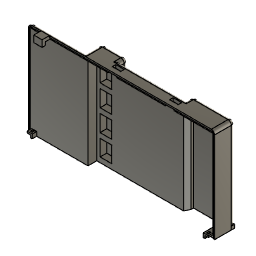
lcd_back (Autodesk Fusion 360 design; units mm, degrees)
Autodesk Fusion 360 part; units mm, degrees
note: some values were not read from the file. Set by a fixed rule: which sketch regions a step uses.
sketch "Szkic1" plane through (0, 0, 0) normal (0, 0, 1) x (1, 0, 0)
  line L0 (0, 0) -> (68.2, 0)
  line L1 (68.2, 0) -> (68.2, 10.6)
  line L2 (68.2, 10.6) -> (176, 10.6)
  line L3 (219, 19.6) -> (219, 23.4)
  line L4 (219, 23.4) -> (62.2, 23.4)
  line L5 (62.2, 23.4) -> (62.2, 3.4)
  line L6 (62.2, 3.4) -> (0, 3.4)
  line L7 (0, 3.4) -> (0, 0)
  circle A0 centre (168, 18.6) radius 1.6
  circle A1 centre (96.5, 18.6) radius 1.6
  line L8 (176, 10.6) -> (176, 19.6)
  line L9 (176, 19.6) -> (219, 19.6)
  dimension "d1" = 62.2
  dimension "d2" = 3.4
  dimension "d3" = 219
  dimension "d4" = 6
  dimension "d5" = 20
  dimension "d6" = 3.2
  dimension "d7" = 3.2
  dimension "d8" = 4.8
  dimension "d9" = 51
  dimension "d10" = 122.5
  dimension "d12" = 12.8
  dimension "d13" = 8
  dimension "d14" = 3.8
  constraint coincident L0.start L7.end
  constraint horizontal L0
  constraint perpendicular L0 L1
  constraint perpendicular L1 L2
  constraint perpendicular L2 L3
  constraint perpendicular L1 L4
  constraint perpendicular L4 L5
  constraint perpendicular L1 L6
  constraint perpendicular L0 L7
  constraint horizontal A0.centre A1.centre
  constraint perpendicular L2 L8
  constraint perpendicular L8 L9
  measures "d1" distance of L5.end L6.end
  measures "d2" distance of L0 L6
  measures "d3" distance of L0.start L3
  measures "d4" distance of L1 L5
  measures "d5" distance of L4 L6
  measures "d6" diameter of A0
  measures "d7" diameter of A1
  measures "d8" distance of L4 A0.centre
  measures "d9" distance of L3 A0.centre
  measures "d10" distance of L3 A1.centre
  measures "d12" distance of L2 L4
  measures "d13" distance of A0.centre L8
  measures "d14" distance of L4 L9
extrude "Wyciągnięcie proste1" add sketch "Szkic1" along normal blind 4
sketch "Szkic2" plane through (0, 0, 4) normal (0, 0, 1) x (-1, 0, 0)
  circle A0 centre (-168, -18.6) radius 1.6
  circle A1 centre (-96.5, -18.6) radius 1.6
  line L0 (-176, -19.6) -> (-219, -19.6)
  line L1 (-219, -19.6) -> (-219, -23.4)
  line L2 (-219, -23.4) -> (-62.2, -23.4)
  line L3 (-62.2, -23.4) -> (-62.2, -3.4)
  line L4 (-62.2, -3.4) -> (0, -3.4)
  line L5 (0, -3.4) -> (0, 0)
  line L6 (0, 0) -> (-68.2, 0)
  line L7 (-68.2, 0) -> (-68.2, -10.6)
  line L8 (-68.2, -10.6) -> (-176, -10.6)
  line L9 (-176, -10.6) -> (-176, -19.6)
  circle A2 centre (-96.5, -18.6) radius 3
  circle A3 centre (-168, -18.6) radius 3
  dimension "d17" = 6
  dimension "d18" = 6
  constraint concentric A1 A2
  constraint concentric A0 A3
  measures "d17" diameter of A2
  measures "d18" diameter of A3
extrude "Wyciągnięcie proste2" cut sketch "Szkic2" against normal blind 2 contours A2 | A3
sketch "Szkic3" plane through (0, 0, 4) normal (0, 0, 1) x (-1, 0, 0)
  circle A0 centre (-96.5, -18.6) radius 3
  circle A1 centre (-168, -18.6) radius 3
  line L0 (-176, -19.6) -> (-219, -19.6)
  line L1 (-219, -19.6) -> (-219, -23.4)
  line L2 (-219, -23.4) -> (-62.2, -23.4)
  line L3 (-62.2, -23.4) -> (-62.2, -3.4)
  line L4 (-62.2, -3.4) -> (0, -3.4)
  line L5 (0, -3.4) -> (0, 0)
  line L6 (0, 0) -> (-68.2, 0)
  line L7 (-68.2, 0) -> (-68.2, -10.6)
  line L8 (-68.2, -10.6) -> (-176, -10.6)
  line L9 (-176, -10.6) -> (-176, -19.6)
  line L10 (0, -3.4) -> (-62.2, -3.4)
  line L11 (-62.2, -23.4) -> (-62.2, -3.4)
  line L12 (-62.2, -23.4) -> (-92.5, -23.4)
  line L13 (-92.5, -14.6) -> (-172, -14.6)
  line L14 (-172, -14.6) -> (-172, -23.4)
  line L15 (-172, -23.4) -> (-219, -23.4)
  line L16 (-219, -23.4) -> (-219, -19.6)
  line L17 (-219, -19.6) -> (-176, -19.6)
  line L18 (-176, -19.6) -> (-176, -10.6)
  line L19 (-176, -10.6) -> (-68.2, -10.6)
  line L20 (-68.2, -10.6) -> (-68.2, 0)
  line L21 (-68.2, 0) -> (0, 0)
  line L22 (0, -3.4) -> (0, 0)
  line L23 (-92.5, -14.6) -> (-92.5, -23.4)
  dimension "d21" = 4
  dimension "d22" = 4
  dimension "d24" = 4
  constraint coincident L4.end L5.start
  constraint coincident L3.end L4.start
  constraint coincident L2.end L3.start
  constraint coincident L2 L12.end
  constraint perpendicular L3 L12
  constraint parallel L8 L13
  constraint coincident L2 L14.end
  constraint perpendicular L2 L14
  constraint coincident L1.end L2.start
  constraint coincident L0.end L1.start
  constraint coincident L0.start L9.end
  constraint coincident L8.end L9.start
  constraint coincident L7.end L8.start
  constraint coincident L6.end L7.start
  constraint coincident L5.end L6.start
  constraint perpendicular L12 L23
  constraint coincident L13.end L14.start
  measures "d21" distance of A0.centre L23
  measures "d22" distance of A1.centre L14
  measures "d24" distance of A0.centre L13
extrude "Wyciągnięcie proste3" add sketch "Szkic3" along normal blind 105.486 contours L0 L1 L2 L3 L4 L5 L6 L7 L8 L9 L10 L11 L12 L13 L14 L15 L16 L17 L18 L19 L20 L21 L22 L23
sketch "Szkic4" plane through (0, 0, 109.486) normal (0, 0, 1) x (-1, 0, 0)
  line L0 (-172, -14.6) -> (-92.5, -14.6)
  line L1 (-92.5, -14.6) -> (-92.5, -23.4)
  line L2 (-92.5, -23.4) -> (-62.2, -23.4)
  line L3 (-62.2, -23.4) -> (-62.2, -3.4)
  line L4 (-62.2, -3.4) -> (0, -3.4)
  line L5 (0, -3.4) -> (0, 0)
  line L6 (0, 0) -> (-68.2, 0)
  line L7 (-68.2, 0) -> (-68.2, -10.6)
  line L8 (-68.2, -10.6) -> (-176, -10.6)
  line L9 (-176, -10.6) -> (-176, -19.6)
  line L10 (-176, -19.6) -> (-219, -19.6)
  line L11 (-219, -19.6) -> (-219, -23.4)
  line L12 (-219, -23.4) -> (-172, -23.4)
  line L13 (-172, -23.4) -> (-172, -14.6)
  line L14 (0, -3.4) -> (-62.2, -3.4)
  line L15 (-62.2, -3.4) -> (-62.2, -23.4)
  line L16 (-62.2, -23.4) -> (-92.5, -23.4)
  line L17 (-92.5, -23.4) -> (-92.5, -14.6)
  line L18 (-92.5, -14.6) -> (-172, -14.6)
  line L19 (-172, -14.6) -> (-172, -23.4)
  line L20 (-172, -23.4) -> (-219, -23.4)
  line L21 (-219, -23.4) -> (-219, -0.0002)
  line L22 (-219, -0.0002) -> (0, 0)
  line L23 (0, 0) -> (0, -3.4)
  constraint coincident L4.end L5.start
  constraint coincident L3.end L4.start
  constraint coincident L2.end L3.start
  constraint coincident L1.end L2.start
  constraint coincident L0.end L1.start
  constraint coincident L0.start L13.end
  constraint coincident L12.end L13.start
  constraint coincident L11.end L12.start
  constraint coincident L5.end L6.start
  constraint perpendicular L21 L22
  constraint perpendicular L22 L23
extrude "Wyciągnięcie proste4" add sketch "Szkic4" along normal blind 4
sketch "Szkic5" plane through (0, 0, 113.486) normal (0, 0, 1) x (-1, 0, 0)
  line L0 (0, 0) -> (-219, -0.0002)
  line L1 (-219, -0.0002) -> (-219, -23.4)
  line L2 (-219, -23.4) -> (-172, -23.4)
  line L3 (-172, -23.4) -> (-172, -14.6)
  line L4 (-172, -14.6) -> (-92.5, -14.6)
  line L5 (-92.5, -14.6) -> (-92.5, -23.4)
  line L6 (-92.5, -23.4) -> (-62.2, -23.4)
  line L7 (-62.2, -23.4) -> (-62.2, -3.4)
  line L8 (-62.2, -3.4) -> (0, -3.4)
  line L9 (0, -3.4) -> (0, 0)
  line L10 (-92.5, -9.2001) -> (-102.7, -9.2001)
  line L11 (-102.7, -9.2001) -> (-102.7, -5.0001)
  line L12 (-102.7, -5.0001) -> (-92.5, -5.0001)
  line L13 (-92.5, -5.0001) -> (-92.5, -9.2001)
  line L14 (-161.8, -9.2001) -> (-172, -9.2001)
  line L15 (-172, -9.2001) -> (-172, -5.0001)
  line L16 (-172, -5.0001) -> (-161.8, -5.0001)
  line L17 (-161.8, -5.0001) -> (-161.8, -9.2001)
  dimension "d29" = 4.2
  dimension "d30" = 10.2
  dimension "d31" = 4.2
  dimension "d32" = 10.2
  dimension "d33" = 5
  dimension "d34" = 5
  constraint horizontal L10
  constraint vertical L11
  constraint horizontal L12
  constraint vertical L13
  constraint horizontal L14
  constraint vertical L15
  constraint horizontal L16
  constraint vertical L17
  constraint vertical L3.end L14.end
  constraint vertical L4.end L10.start
  measures "d29" distance of L10.start L12.end
  measures "d30" distance of L10.start L10.end
  measures "d31" distance of L14.end L15.end
  measures "d32" distance of L14.start L14.end
  measures "d33" distance of L0 L12
  measures "d34" distance of L0 L16
extrude "Wyciągnięcie proste5" cut sketch "Szkic5" against normal blind 5 contours L10 L11 L12 L13 | L14 L15 L16 L17
sketch "Szkic6" plane through (0, 0, 109.486) normal (0, 0, -1) x (1, 0, 0)
  line L0 (102.7, -5.0001) -> (102.7, -9.2001)
  line L1 (102.7, -9.2001) -> (92.5, -9.2001)
  line L2 (92.5, -9.2001) -> (92.5, -5.0001)
  line L3 (92.5, -5.0001) -> (102.7, -5.0001)
  line L4 (172, -5.0001) -> (172, -9.2001)
  line L5 (172, -9.2001) -> (161.8, -9.2001)
  line L6 (161.8, -9.2001) -> (161.8, -5.0001)
  line L7 (161.8, -5.0001) -> (172, -5.0001)
  line L8 (68.2, -0.0001) -> (68.2, -10.6)
  line L9 (68.2, -10.6) -> (176, -10.6)
  line L10 (176, -10.6) -> (176, -19.6)
  line L11 (176, -19.6) -> (219, -19.6)
  line L12 (219, -19.6) -> (219, -0.0002)
  line L13 (219, -0.0002) -> (68.2, -0.0001)
  line L14 (92.5, -5.0001) -> (102.7, -5.0001)
  line L15 (102.7, -5.0001) -> (102.7, -0.0001)
  line L16 (102.7, -0.0001) -> (92.5, -0.0001)
  line L17 (92.5, -0.0001) -> (92.5, -5.0001)
  line L18 (161.8, -5.0001) -> (172, -5.0001)
  line L19 (172, -5.0001) -> (172, -0.0001)
  line L20 (172, -0.0001) -> (161.8, -0.0001)
  line L21 (161.8, -0.0001) -> (161.8, -5.0001)
  constraint horizontal L14
  constraint vertical L15
  constraint horizontal L16
  constraint vertical L17
  constraint coincident L2.end L3.start
  constraint horizontal L18
  constraint vertical L19
  constraint horizontal L20
  constraint vertical L21
  constraint coincident L6.end L7.start
  constraint coincident L0.start L3.end
  constraint coincident L13 L15.end
  constraint coincident L13 L19.end
  constraint coincident L4.start L19
extrude "Wyciągnięcie proste6" cut sketch "Szkic6" against normal blind 2 contours L3 L13 L14 L15 L16 L17 | L7 L13 L18 L19 L20 L21
sketch "Szkic7" plane through (0, 0, 0) normal (-1, 0, 0) x (0, -1, 0)
  line L0 (-3.4, 0) -> (0, 0)
  line L1 (0, 0) -> (0, 109.486)
  line L2 (0, 109.486) -> (0, 113.486)
  line L3 (0, 113.486) -> (-3.4, 113.486)
  line L4 (-3.4, 113.486) -> (-3.4, 0)
  line L5 (-3.4, 113.486) -> (0, 113.486)
  line L6 (0, 113.486) -> (0, 0)
  line L7 (0, 0) -> (-3.4, 0)
  line L8 (-3.4, 0) -> (-3.4, 113.486)
  constraint horizontal L5
  constraint vertical L6
  constraint horizontal L7
  constraint vertical L8
  constraint coincident L0.end L1.start
  constraint coincident L3.end L4.start
extrude "Wyciągnięcie proste7" add sketch "Szkic7" along normal blind 2.8
sketch "Szkic8" plane through (219, 0.0002, 0) normal (1, 0.000001, 0) x (-0.000001, 1, 0)
  line L0 (19.5998, 0) -> (23.3998, 0)
  line L1 (23.3998, 0) -> (23.3998, 113.486)
  line L2 (23.3998, 113.486) -> (0, 113.486)
  line L3 (0, 113.486) -> (0, 109.486)
  line L4 (0, 109.486) -> (19.5998, 109.486)
  line L5 (19.5998, 109.486) -> (19.5998, 0)
  line L6 (23.3998, 113.486) -> (0, 113.486)
  line L7 (0, 113.486) -> (0, 0)
  line L8 (0, 0) -> (23.3998, 0)
  line L9 (23.3998, 0) -> (23.3998, 113.486)
  constraint horizontal L6
  constraint vertical L7
  constraint horizontal L8
  constraint vertical L9
  constraint coincident L7.end L8.start
  constraint coincident L1.end L2.start
extrude "Wyciągnięcie proste8" add sketch "Szkic8" along normal blind 2.8
sketch "Szkic9" plane through (0, 0, 113.486) normal (0, 0, 1) x (-1, 0, 0)
  line L0 (-102.7, -9.2001) -> (-102.7, -5.0001)
  line L1 (-102.7, -5.0001) -> (-92.5, -5.0001)
  line L2 (-92.5, -5.0001) -> (-92.5, -9.2001)
  line L3 (-92.5, -9.2001) -> (-102.7, -9.2001)
  line L4 (-172, -9.2001) -> (-172, -5.0001)
  line L5 (-172, -5.0001) -> (-161.8, -5.0001)
  line L6 (-161.8, -5.0001) -> (-161.8, -9.2001)
  line L7 (-161.8, -9.2001) -> (-172, -9.2001)
  line L8 (0, 0) -> (-221.8, -0.0002)
  line L9 (-221.8, -0.0002) -> (-221.8, -23.4)
  line L10 (-221.8, -23.4) -> (-219, -23.4)
  line L11 (-219, -23.4) -> (-172, -23.4)
  line L12 (-172, -23.4) -> (-172, -14.6)
  line L13 (-172, -14.6) -> (-92.5, -14.6)
  line L14 (-92.5, -14.6) -> (-92.5, -23.4)
  line L15 (-92.5, -23.4) -> (-62.2, -23.4)
  line L16 (-62.2, -23.4) -> (-62.2, -3.4)
  line L17 (-62.2, -3.4) -> (2.8, -3.4)
  line L18 (2.8, -3.4) -> (2.8, 0)
  line L19 (2.8, 0) -> (0, 0)
  line L20 (-12.2, 0) -> (-22.2, 0)
  line L21 (-22.2, 0) -> (-22.2, 9.4)
  line L22 (-22.2, 9.4) -> (-12.2, 9.4)
  line L23 (-12.2, 9.4) -> (-12.2, 0)
  dimension "d43" = 9.4
  dimension "d44" = 10
  dimension "d45" = 15
  constraint horizontal L20
  constraint vertical L21
  constraint horizontal L22
  constraint vertical L23
  constraint coincident L8 L20.end
  measures "d43" distance of L8 L22
  measures "d44" distance of L21 L23
  measures "d45" distance of L18 L23
extrude "Wyciągnięcie proste9" add sketch "Szkic9" against normal blind 4 contours L8 L20 L21 L22 L23
sketch "Szkic10" plane through (0, 0, 109.486) normal (0, 0, -1) x (1, 0, 0)
  line L0 (22.2, 9.4) -> (12.2, 9.4)
  line L1 (12.2, 9.4) -> (12.2, 0)
  line L2 (12.2, 0) -> (22.2, 0)
  line L3 (22.2, 0) -> (22.2, 9.4)
  line L4 (12.2, 9.4) -> (22.2, 9.4)
  line L5 (22.2, 9.4) -> (22.2, 5.4)
  line L6 (22.2, 5.4) -> (12.2, 5.4)
  line L7 (12.2, 5.4) -> (12.2, 9.4)
  dimension "d48" = 4
  constraint horizontal L4
  constraint vertical L5
  constraint horizontal L6
  constraint vertical L7
  constraint coincident L3 L5.end
  constraint coincident L0.end L1.start
  measures "d48" distance of L4 L6
extrude "Wyciągnięcie proste10" add sketch "Szkic10" along normal blind 4 contours L0 L1 L3 L4 L5 L6 L7
sketch "Szkic12" plane through (219, 0.0002, 0) normal (-1, -0.000001, 0) x (0.000001, -1, 0)
  line L0 (-19.5998, 109.486) -> (-19.5998, 0)
  line L1 (-19.5998, 0) -> (0, 0)
  line L2 (0, 0) -> (0, 109.486)
  line L3 (0, 109.486) -> (-19.5998, 109.486)
  line L4 (0, 0) -> (-19.5998, 0)
  line L5 (-19.5998, 0) -> (-19.5998, 5)
  line L6 (-19.5998, 5) -> (0, 5)
  line L7 (0, 5) -> (0, 0)
  dimension "d58" = 5
  constraint horizontal L4
  constraint vertical L5
  constraint horizontal L6
  constraint vertical L7
  constraint coincident L0 L5.end
  constraint coincident L1.end L2.start
  measures "d58" distance of L4 L6
extrude "Wyciągnięcie proste12" add sketch "Szkic12" along normal blind 6.3 contours L0 L1 L2 L4 L5 L6 L7
sketch "Szkic13" plane through (0, 0, 0) normal (0.000001, -1, 0) x (1, 0.000001, 0)
  line L0 (22.2, 113.486) -> (22.2, 109.486)
  line L1 (22.2, 109.486) -> (68.2, 109.486)
  line L2 (68.2, 109.486) -> (92.5, 109.486)
  line L3 (92.5, 109.486) -> (92.5, 111.486)
  line L4 (92.5, 111.486) -> (102.7, 111.486)
  line L5 (102.7, 111.486) -> (102.7, 109.486)
  line L6 (102.7, 109.486) -> (161.8, 109.486)
  line L7 (161.8, 109.486) -> (161.8, 111.486)
  line L8 (161.8, 111.486) -> (172, 111.486)
  line L9 (172, 111.486) -> (172, 109.486)
  line L10 (172, 109.486) -> (219, 109.486)
  line L11 (219, 109.486) -> (219, 5)
  line L12 (219, 5) -> (212.7, 5)
  line L13 (212.7, 5) -> (212.7, 0)
  line L14 (212.7, 0) -> (221.8, 0)
  line L15 (221.8, 0) -> (221.8, 113.486)
  line L16 (221.8, 113.486) -> (22.2, 113.486)
  line L17 (212.7, 0) -> (218.9, 0)
  line L18 (218.9, 0) -> (218.9, 5)
  line L19 (218.9, 5) -> (212.7, 5)
  line L20 (212.7, 5) -> (212.7, 0)
  dimension "d61" = 0.1
  constraint horizontal L17
  constraint vertical L18
  constraint horizontal L19
  constraint vertical L20
  constraint coincident L12 L18.end
  constraint coincident L13.end L14.start
  measures "d61" distance of L11 L18
extrude "Wyciągnięcie proste13" add sketch "Szkic13" along normal blind 5.4 contours L12 L13 L14 L17 L18 L19 L20
sketch "Szkic14" plane through (218.9, 0.0002, 0) normal (1, 0.000001, 0) x (-0.000001, 1, 0)
  line L0 (0, 0) -> (0, 5)
  line L1 (0, 5) -> (-5.4, 5)
  line L2 (-5.4, 5) -> (-5.4, 0)
  line L3 (-5.4, 0) -> (0, 0)
  line L4 (-5.4, 0) -> (0, 0)
  line L5 (0, 0) -> (0, 3.1)
  line L6 (0, 3.1) -> (-5.4, 3.1)
  line L7 (-5.4, 3.1) -> (-5.4, 0)
  dimension "d64" = 3.1
  constraint horizontal L4
  constraint vertical L5
  constraint horizontal L6
  constraint vertical L7
  constraint coincident L0 L5.end
  constraint coincident L2.end L3.start
  measures "d64" distance of L2.end L6.end
extrude "Wyciągnięcie proste14" cut sketch "Szkic14" against normal blind 4.2 contours L0 L2 L3 L4 L5 L6 L7
sketch "Szkic15" plane through (0, 0, 5) normal (0, 0, 1) x (-1, 0, 0)
  line L0 (-219, -0.0002) -> (-219, -19.6)
  line L1 (-219, -19.6) -> (-212.7, -19.6)
  line L2 (-212.7, -19.6) -> (-212.7, 5.3998)
  line L3 (-212.7, 5.3998) -> (-218.9, 5.3998)
  line L4 (-218.9, 5.3998) -> (-218.9, -0.0002)
  line L5 (-218.9, -0.0002) -> (-219, -0.0002)
  line L6 (-214.7, 0.1998) -> (-216.9, 0.1998)
  line L7 (-216.9, 0.1998) -> (-216.9, 3.3998)
  line L8 (-216.9, 3.3998) -> (-214.7, 3.3998)
  line L9 (-214.7, 3.3998) -> (-214.7, 0.1998)
  dimension "d67" = 2.2
  dimension "d68" = 3.2
  dimension "d69" = 2
  dimension "d70" = 2
  constraint horizontal L6
  constraint vertical L7
  constraint horizontal L8
  constraint vertical L9
  measures "d67" distance of L6.start L6.end
  measures "d68" distance of L6.end L7.end
  measures "d69" distance of L4 L7
  measures "d70" distance of L3 L8
extrude "Wyciągnięcie proste15" cut sketch "Szkic15" against normal blind 10 contours L6 L7 L8 L9
sketch "Szkic16" plane through (0, 0, 0) normal (0, -1, 0) x (1, 0, 0)
  line L0 (-2.8, 0) -> (68.2, 0)
  line L1 (68.2, 0) -> (68.2, 109.486)
  line L2 (68.2, 109.486) -> (22.2, 109.486)
  line L3 (22.2, 109.486) -> (12.2, 109.486)
  line L4 (12.2, 109.486) -> (0, 109.486)
  line L5 (0, 109.486) -> (0, 113.486)
  line L6 (0, 113.486) -> (-2.8, 113.486)
  line L7 (-2.8, 113.486) -> (-2.8, 0)
  line L8 (0.1, 0) -> (6.3, 0)
  line L9 (6.3, 0) -> (6.3, 5)
  line L10 (6.3, 5) -> (0.1, 5)
  line L11 (0.1, 5) -> (0.1, 0)
  dimension "d73" = 2.9
  dimension "d74" = 5
  dimension "d75" = 6.2
  constraint horizontal L8
  constraint vertical L9
  constraint horizontal L10
  constraint vertical L11
  constraint coincident L0 L8.start
  measures "d73" distance of L7 L11
  measures "d74" distance of L8.end L9.end
  measures "d75" distance of L9.end L10.end
extrude "Wyciągnięcie proste16" add sketch "Szkic16" along normal blind 5.4 contours L0 L8 L9 L10 L11
sketch "Szkic18" plane through (0.1, 0, 0) normal (-1, 0, 0) x (0, -1, 0)
  line L0 (0, 5) -> (0, 0)
  line L1 (0, 0) -> (5.4, 0)
  line L2 (5.4, 0) -> (5.4, 5)
  line L3 (5.4, 5) -> (0, 5)
  line L4 (5.4, 0) -> (-0.0002, 0)
  line L5 (-0.0002, 0) -> (-0.0002, 3.1)
  line L6 (-0.0002, 3.1) -> (5.4, 3.1)
  line L7 (5.4, 3.1) -> (5.4, 0)
  point P0 (-0.0002, 3.1)
  dimension "d80" = 3.1
  constraint horizontal L4
  constraint vertical L5
  constraint horizontal L6
  constraint vertical L7
  constraint coincident L1.end L2.start
  constraint coincident P0 L5.end
  measures "d80" distance of L1.end L6.end
extrude "Wyciągnięcie proste17" cut sketch "Szkic18" against normal blind 4.2 contours L0 L1 L2 L4 L5 L6 L7
sketch "Szkic19" plane through (0, 0, 5) normal (0, 0, 1) x (-1, 0, 0)
  line L0 (-6.3, 0) -> (-0.1, 0)
  line L1 (-0.1, 0) -> (-0.1, 5.4)
  line L2 (-0.1, 5.4) -> (-6.3, 5.4)
  line L3 (-6.3, 5.4) -> (-6.3, 0)
  line L4 (-2.1, 0.2) -> (-4.3, 0.2)
  line L5 (-4.3, 0.2) -> (-4.3, 3.4)
  line L6 (-4.3, 3.4) -> (-2.1, 3.4)
  line L7 (-2.1, 3.4) -> (-2.1, 0.2)
  dimension "d83" = 2.2
  dimension "d84" = 3.2
  dimension "d85" = 2
  dimension "d86" = 2
  constraint horizontal L4
  constraint vertical L5
  constraint horizontal L6
  constraint vertical L7
  measures "d83" distance of L4.start L4.end
  measures "d84" distance of L4.end L5.end
  measures "d85" distance of L2 L6
  measures "d86" distance of L1 L7
extrude "Wyciągnięcie proste18" cut sketch "Szkic19" against normal blind 10 contours L4 L5 L6 L7
sketch "Szkic20" plane through (0, 0, 0) normal (0.000001, -1, 0) x (1, 0.000001, 0)
  line L0 (218.9, 5) -> (218.9, 3.1)
  line L1 (218.9, 3.1) -> (214.7, 3.1)
  line L2 (214.7, 3.1) -> (214.7, 0)
  line L3 (214.7, 0) -> (221.8, 0)
  line L4 (221.8, 0) -> (221.8, 113.486)
  line L5 (221.8, 113.486) -> (22.2, 113.486)
  line L6 (22.2, 113.486) -> (22.2, 109.486)
  line L7 (22.2, 109.486) -> (68.2, 109.486)
  line L8 (68.2, 109.486) -> (92.5, 109.486)
  line L9 (92.5, 109.486) -> (92.5, 111.486)
  line L10 (92.5, 111.486) -> (102.7, 111.486)
  line L11 (102.7, 111.486) -> (102.7, 109.486)
  line L12 (102.7, 109.486) -> (161.8, 109.486)
  line L13 (161.8, 109.486) -> (161.8, 111.486)
  line L14 (161.8, 111.486) -> (172, 111.486)
  line L15 (172, 111.486) -> (172, 109.486)
  line L16 (172, 109.486) -> (219, 109.486)
  line L17 (219, 109.486) -> (219, 5)
  line L18 (219, 5) -> (218.9, 5)
  line L19 (22.2, 113.486) -> (221.8, 113.486)
  line L20 (221.8, 113.486) -> (221.8, 0)
  line L21 (221.8, 0) -> (220.55, 0)
  line L22 (220.55, 0) -> (220.55, 110.136)
  line L23 (219.05, 111.636) -> (22.2, 111.636)
  line L24 (22.2, 111.636) -> (22.2, 113.486)
  arc A0 (220.55, 110.136) -> (219.05, 111.636) centre (219.05, 110.136) ccw
  dimension "d89" = 1.85
  dimension "d90" = 1.25
  dimension "d112" = 3
  constraint coincident L5.end L6.start
  constraint coincident L4.end L5.start
  constraint coincident L3.end L4.start
  constraint coincident L3 L21.end
  constraint perpendicular L4 L21
  constraint perpendicular L19 L22
  constraint coincident L6 L23.end
  constraint perpendicular L23 L24
  constraint tangent L22 A0
  constraint tangent L23 A0
  measures "d89" distance of L19 L23
  measures "d90" distance of L20 L22
  measures "d112" diameter of A0
extrude "Wyciągnięcie proste19" add sketch "Szkic20" along normal blind 0.8 contours L3 L4 L5 L6 L19 L20 L21 L22 L23 L24 A0
sketch "Szkic21" plane through (0, 0, 0) normal (0.000001, -1, 0) x (1, 0.000001, 0)
  line L0 (12.2, 109.486) -> (12.2, 113.486)
  line L1 (12.2, 113.486) -> (0, 113.486)
  line L2 (0, 113.486) -> (0, 109.486)
  line L3 (0, 109.486) -> (12.2, 109.486)
  line L4 (0, 113.486) -> (12.2, 113.486)
  line L5 (12.2, 113.486) -> (12.2, 111.636)
  line L6 (12.2, 111.636) -> (0, 111.636)
  line L7 (0, 111.636) -> (0, 113.486)
  dimension "d93" = 1.85
  constraint horizontal L4
  constraint vertical L5
  constraint horizontal L6
  constraint vertical L7
  constraint coincident L0 L5.end
  constraint coincident L1.end L2.start
  measures "d93" distance of L4 L6
extrude "Wyciągnięcie proste20" add sketch "Szkic21" along normal blind 0.8 contours L0 L1 L2 L4 L5 L6 L7
sketch "Szkic22" plane through (0, 0, 0) normal (0, -1, 0) x (1, 0, 0)
  line L0 (6.3, 5) -> (6.3, 0)
  line L1 (6.3, 0) -> (68.2, 0)
  line L2 (68.2, 0) -> (68.2, 109.486)
  line L3 (68.2, 109.486) -> (22.2, 109.486)
  line L4 (22.2, 109.486) -> (12.2, 109.486)
  line L5 (12.2, 109.486) -> (0, 109.486)
  line L6 (0, 109.486) -> (0, 111.636)
  line L7 (0, 111.636) -> (0, 113.486)
  line L8 (0, 113.486) -> (-2.8, 113.486)
  line L9 (-2.8, 113.486) -> (-2.8, 0)
  line L10 (-2.8, 0) -> (4.3, 0)
  line L11 (4.3, 0) -> (4.3, 3.1)
  line L12 (4.3, 3.1) -> (0.1, 3.1)
  line L13 (0.1, 3.1) -> (0.1, 5)
  line L14 (0.1, 5) -> (6.3, 5)
  line L15 (-1.55, 0) -> (-2.8, 0)
  line L16 (-2.8, 0) -> (-2.8, 113.486)
  line L17 (0, 113.486) -> (-2.8, 113.486)
  line L18 (0, 113.486) -> (0, 111.636)
  line L19 (0, 111.636) -> (-0.05, 111.636)
  line L20 (-1.55, 110.136) -> (-1.55, 0)
  arc A0 (0, 111.6352) -> (-1.55, 110.136) centre (-0.05, 110.136) ccw
  dimension "d96" = 1.25
  dimension "d113" = 3
  constraint coincident L10 L15.start
  constraint coincident L9.end L10.start
  constraint perpendicular L9 L15
  constraint coincident L8.end L9.start
  constraint coincident L7.end L8.start
  constraint coincident L6.end L7.start
  constraint perpendicular L7 L19
  constraint perpendicular L19 L20
  constraint tangent L19 A0
  constraint tangent L20 A0
  constraint coincident L19.end A0
  constraint coincident L6 A0.start
  measures "d96" distance of L16 L20
  measures "d113" diameter of A0
extrude "Wyciągnięcie proste21" add sketch "Szkic22" along normal blind 0.8 contours L7 L8 L9 L10 L15 L16 L17 L18 L19 L20 A0
fillet "Zaokrąglenie3" radius 4 15 edges at (221.8, 11.3001, 113.486) (221.8, 23.4, 56.743) (220.4, 23.4, 113.486) (195.5, 23.4, 113.486) (172, 19, 113.486) (132.25, 14.6, 113.486) (172, 23.4, 58.743) (92.5, 23.4, 58.743) (92.5, 19, 113.486) (77.35, 23.4, 113.486) (62.2, 23.4, 56.743) (-2.8, 1.3, 113.486) (-2.8, 3.4, 56.743) (29.7, 3.4, 113.486) (62.2, 13.4, 113.486)
sketch "Szkic24" plane through (0, 0, 0) normal (0, 0, -1) x (1, 0, 0)
  circle A0 centre (168, -18.6) radius 1.6
  circle A1 centre (96.5, -18.6) radius 1.6
  arc A2 (217.8, -23.4) -> (221.8, -19.4) centre (217.8, -19.4) ccw
  line L0 (221.8, -19.4) -> (221.8, 0.7998)
  line L1 (221.8, 0.7998) -> (220.55, 0.7998)
  line L2 (220.55, 0.7998) -> (220.55, -0.0002)
  line L3 (220.55, -0.0002) -> (214.7, -0.0002)
  line L4 (214.7, -0.0002) -> (214.7, 5.3998)
  line L5 (214.7, 5.3998) -> (212.7, 5.3998)
  line L6 (212.7, 5.3998) -> (212.7, -19.6)
  line L7 (212.7, -19.6) -> (176, -19.6)
  line L8 (176, -19.6) -> (176, -10.6)
  line L9 (176, -10.6) -> (68.2, -10.6)
  line L10 (68.2, -10.6) -> (68.2, 0)
  line L11 (68.2, 0) -> (6.3, 0)
  line L12 (6.3, 0) -> (6.3, 5.4)
  line L13 (6.3, 5.4) -> (4.3, 5.4)
  line L14 (4.3, 5.4) -> (4.3, 0)
  line L15 (4.3, 0) -> (-1.55, 0)
  line L16 (-1.55, 0) -> (-1.55, 0.8)
  line L17 (-1.55, 0.8) -> (-2.8, 0.8)
  line L18 (-2.8, 0.8) -> (-2.8, 0.6)
  arc A3 (-2.8, 0.6) -> (1.2, -3.4) centre (1.2, 0.6) ccw
  line L19 (1.2, -3.4) -> (62.2, -3.4)
  line L20 (62.2, -3.4) -> (62.2, -19.4)
  arc A4 (62.2, -19.4) -> (66.2, -23.4) centre (66.2, -19.4) ccw
  line L21 (66.2, -23.4) -> (217.8, -23.4)
  line L22 (1.2, -3.4) -> (-2.8, -3.4)
  line L23 (-2.8, -3.4) -> (-2.8, 0.8)
  line L24 (-2.8, 0.8) -> (1.2, -3.4)
  line L25 (66.2, -23.4) -> (62.2, -23.4)
  line L26 (62.2, -23.4) -> (62.2, -19.4)
  line L27 (62.2, -19.4) -> (66.2, -23.4)
  line L28 (217.8, -23.4) -> (221.8, -23.4)
  line L29 (221.8, -23.4) -> (221.8, -19.4)
  line L30 (221.8, -19.4) -> (217.8, -23.4)
  constraint horizontal L22
  constraint vertical L23
  constraint coincident L17.end L18.start
  constraint coincident A3.end L19.start
  constraint horizontal L25
  constraint vertical L26
  constraint coincident L20.end A4.start
  constraint coincident A4.end L21.start
  constraint horizontal L28
  constraint vertical L29
  constraint coincident A2.start L21.end
  constraint coincident A2.end L0.start
extrude "Wyciągnięcie proste23" add sketch "Szkic24" against normal blind 4 contours A2 L28 L29 | A4 L25 L26 | A3 L22 L23
sketch "Szkic25" plane through (0, 10.6, 0) normal (0, -1, 0) x (1, 0, 0)
  line L0 (68.2, 0) -> (176, 0)
  line L1 (176, 0) -> (176, 109.486)
  line L2 (176, 109.486) -> (68.2, 109.486)
  line L3 (68.2, 109.486) -> (68.2, 0)
  line L4 (72.2, 103.486) -> (86.2, 103.486)
  line L5 (86.2, 103.486) -> (86.2, 83.486)
  line L6 (86.2, 83.486) -> (72.2, 83.486)
  line L7 (72.2, 83.486) -> (72.2, 103.486)
  line L8 (72.2, 77.486) -> (86.2, 77.486)
  line L9 (86.2, 77.486) -> (86.2, 57.486)
  line L10 (86.2, 57.486) -> (72.2, 57.486)
  line L11 (72.2, 57.486) -> (72.2, 77.486)
  line L12 (72.2, 51.486) -> (86.2, 51.486)
  line L13 (86.2, 51.486) -> (86.2, 31.486)
  line L14 (86.2, 31.486) -> (72.2, 31.486)
  line L15 (72.2, 31.486) -> (72.2, 51.486)
  line L16 (72.2, 25.486) -> (86.2, 25.486)
  line L17 (86.2, 25.486) -> (86.2, 6)
  line L18 (86.2, 6) -> (72.2, 6)
  line L19 (72.2, 6) -> (72.2, 25.486)
  dimension "d114" = 4
  dimension "d115" = 6
  dimension "d116" = 14
  dimension "d117" = 6
  dimension "d118" = 6
  dimension "d119" = 6
  dimension "d120" = 6
  dimension "d121" = 20
  dimension "d122" = 20
  dimension "d123" = 20
  constraint horizontal L4
  constraint vertical L5
  constraint horizontal L6
  constraint vertical L7
  constraint horizontal L8
  constraint vertical L9
  constraint horizontal L10
  constraint vertical L11
  constraint horizontal L12
  constraint vertical L13
  constraint horizontal L14
  constraint vertical L15
  constraint horizontal L16
  constraint vertical L17
  constraint horizontal L18
  constraint vertical L19
  constraint vertical L6.end L8.start
  constraint vertical L10.end L12.start
  constraint vertical L14.end L16.start
  constraint vertical L13.end L16.end
  constraint vertical L9.end L12.end
  constraint vertical L5.end L8.end
  measures "d114" distance of L3 L7
  measures "d115" distance of L2 L4
  measures "d116" distance of L5 L7
  measures "d117" distance of L6 L8
  measures "d118" distance of L10 L12
  measures "d119" distance of L14 L16
  measures "d120" distance of L0 L18
  measures "d121" distance of L4.end L5.end
  measures "d122" distance of L8.end L9.end
  measures "d123" distance of L12.end L13.end
extrude "Wyciągnięcie proste24" cut sketch "Szkic25" against normal blind 8 contours L4 L5 L6 L7 | L8 L9 L10 L11 | L12 L13 L14 L15 | L16 L17 L18 L19
chamfer "Fazowanie1" distance 3 distance2 6 1 edges at (176, 10.6, 54.743) measured on face at (146.0667, 10.6, 55.6573)
